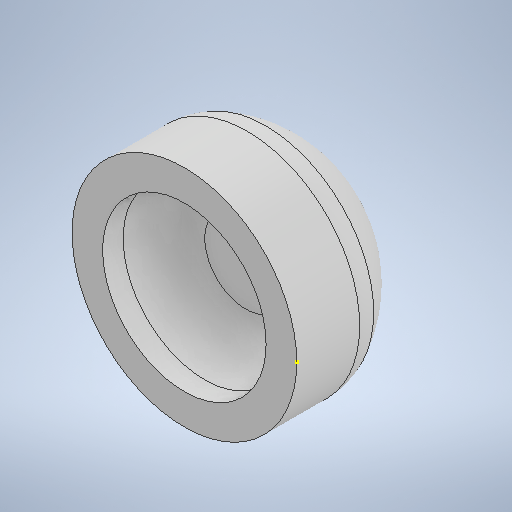
# Autodesk Inventor part: Part1 finger tip(pinky)
Saved by Autodesk Inventor 2025 (Build 290162000, 162)
## iProperties
Created: 2025-10-18
Part Number: Part1 finger tip(pinky)
Material: Generic
Document SubType Name: Modeling
Designer: abdul
Density: 1 g/cm^3
Appearance: Default
Author: abdul
Autodesk Inventor part; units mm, degrees
ref_plane "YZ Plane" through (0, 0, 0) normal (1, 0, 0) x (0, 1, 0)
ref_plane "XZ Plane" through (0, 0, 0) normal (0, 1, 0) x (-1, 0, 0)
ref_plane "XY Plane" through (0, 0, 0) normal (0, 0, 1) x (1, 0, 0)
sketch "Sketch1" plane through (0, 0, 0) normal (0, 1, 0) x (-1, 0, 0)
  line L0 (5.5, 0) -> (0, 0)
  line L1 (0, 0) -> (0, -3.5)
  line L2 (5.5, 0) -> (5.5, -7)
  arc A0 (0, -3.5) -> (5.5, -7) centre (5.1284, -1.5126) ccw
  dimension "d2" = 3.5
  dimension "d6" = 7
  dimension "d7" = 5.5
  dimension "d8" = 5.5
  dimension "d9" = 1.5126
  constraints: 6 end point, 2 point on circle, 2 vertical, 1 centre point
  measures "d2" distance of L0.end L1.end
  measures "d6" distance of L0.start L2.end
  measures "d7" radius of A0
  measures "d8" distance between parallel lines of L1 L2
  measures "d9" distance from line of A0.centre L0
revolve "Revolution1" add sketch "Sketch1" angle 360 about axis through (-5.5, 0, 0) along (0, 0, -1)
fillet "Fillet1" radius 2 1 edges at (-11, 0, -3.5)
sketch "Sketch2" plane through (-5.5, 0, 0) normal (0, 0, 1) x (1, 0, 0)
  point P0 (5.5, 0)
sketch "Sketch3" plane through (-5.5, 0, 0) normal (0, 0, 1) x (1, 0, 0)
  circle A0 centre (0, 0) radius 4
  circle A1 centre (0, 0) radius 5.5 projected
  point P0 (5.5, 0)
  dimension "d12" = 8
  dimension "d13" = 1.5
  constraints: 1 centre point, 1 horizontal alignment
  measures "d12" diameter of A0
extrude "Extrusion1" cut sketch "Sketch3" against normal blind 3 contours A0
fillet "Fillet2" radius 2 1 edges at (-9.5, 0, -3)
body "Solid1"
